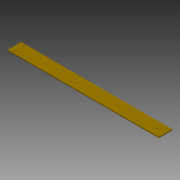
# Autodesk Inventor part: X Rail
Saved by Autodesk Inventor 2013 (Build 170138000, 138)
## iProperties
Created: 2017-01-25
Part Number: X Rail
Material: Generic
Document SubType Name: Modeling
Designer: Herman de Vries
Density: 1 g/cm^3
Author: Herman de Vries
Autodesk Inventor part; units mm, degrees
ref_plane "YZ Plane" through (0, 0, 0) normal (1, 0, 0) x (0, 1, 0)
ref_plane "XZ Plane" through (0, 0, 0) normal (0, 1, 0) x (-1, 0, 0)
ref_plane "XY Plane" through (0, 0, 0) normal (0, 0, 1) x (1, 0, 0)
sketch "Sketch1" plane through (0, 0, 0) normal (1, 0, 0) x (0, 1, 0)
  line L0 (0, 0) -> (50, 0)
  line L1 (50, 0) -> (50, 3)
  line L2 (50, 3) -> (0, 3)
  line L3 (0, 3) -> (0, 0)
  dimension "d0" = 50
  dimension "d1" = 3
  constraints: 8 end point, 2 parallel, 1 horizontal, 1 perpendicular
  measures "d0" distance of L2.end L1.end
  measures "d1" distance of L1.end L0.end
extrude "Extrusion1" add sketch "Sketch1" along normal blind 560
sketch "Sketch2" plane through (0, 0, 3) normal (0, 0, 1) x (1, 0, 0)
  line L0 (0, 0) -> (560, 0) projected
  line L1 (0, 50) -> (560, 50) projected
  line L2 (0, 50) -> (0, 0) projected
  line L3 (560, 50) -> (560, 0) projected
  line L4 (17.5, 41) -> (49.5, 41) construction
  line L5 (49.5, 41) -> (49.5, 9) construction
  line L6 (49.5, 9) -> (17.5, 9) construction
  line L7 (17.5, 9) -> (17.5, 41) construction
  circle A0 centre (17.5, 41) radius 1.5
  circle A1 centre (49.5, 41) radius 1.5
  circle A2 centre (49.5, 9) radius 1.5
  circle A3 centre (17.5, 9) radius 1.5
  circle A4 centre (530, 25) radius 1.5
  point P0 (560, 25)
  point P1 (17.5, 25)
  point P2 (0, 25)
  dimension "d12" = 32
  dimension "d13" = 32
  dimension "d14" = 17.5
  dimension "d15" = 3
  dimension "d16" = 3
  dimension "d17" = 3
  dimension "d18" = 3
  dimension "d19" = 3
  dimension "d20" = 30
  constraints: 8 end point, 5 centre point, 4 coincident, 3 midpoint, 2 parallel, 1 horizontal, 1 horizontal alignment, 1 perpendicular
  measures "d12" distance of L5.end L6.end
  measures "d13" distance of L4.end L5.end
  measures "d14" distance between parallel lines of L2 L7
  measures "d15" diameter of A0
  measures "d16" diameter of A1
  measures "d17" diameter of A2
  measures "d18" diameter of A3
  measures "d19" diameter of A4
  measures "d20" distance from line of A4.centre L3
extrude "Extrusion2" cut sketch "Sketch2" against normal blind 10 contours A0 | A1 | A2 | A3 | A4
body "Solid1"
